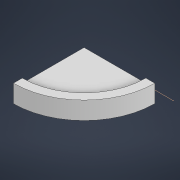
# Autodesk Inventor part: McCrea_zakruta_walle
Saved by Autodesk Inventor 2022 (Build 260153000, 153)
## iProperties
Created: 2022-02-12
Part Number: McCrea_zakruta_walle
Material: Generic
Document SubType Name: Modeling
Designer: MatusBarany
Density: 1 g/cm^3
Appearance: Default
Author: MatusBarany
Autodesk Inventor part; units mm, degrees
ref_plane "YZ Plane" through (0, 0, 0) normal (1, 0, 0) x (0, 1, 0)
ref_plane "XZ Plane" through (0, 0, 0) normal (0, 1, 0) x (-1, 0, 0)
ref_plane "XY Plane" through (0, 0, 0) normal (0, 0, 1) x (1, 0, 0)
sketch "Sketch1" plane through (0, 0, 0) normal (0, 1, 0) x (-1, 0, 0)
  arc A0 (740.7704, 834.1348) -> (40.7704, 134.1348) centre (740.7704, 134.1348) ccw
  line L0 (740.7704, 134.1348) -> (40.7704, 134.1348)
  line L1 (740.7704, 134.1348) -> (740.7704, 834.1348)
  line L2 (909.7653, 0) -> (-273.1993, 0) projected
  dimension "d2" = 1400
  constraints: 4 end point, 2 point on circle, 1 centre point, 1 parallel, 1 perpendicular
  measures "d2" diameter of A0
extrude "Extrusion1" add sketch "Sketch1" along normal blind 150
sketch "Sketch2" plane through (0, 0, 0) normal (0, -1, 0) x (1, 0, 0)
  arc A0 (-40.7704, 134.1348) -> (-740.7704, 834.1348) centre (-740.7704, 134.1348) ccw projected
  line L0 (-740.7704, 134.1348) -> (-740.7704, 834.1348) projected
  line L1 (-40.7704, 134.1348) -> (-740.7704, 134.1348) projected
  arc A1 (59.2296, 134.1348) -> (-740.7704, 934.1348) centre (-740.7704, 134.1348) ccw
  arc A2 (-40.7704, 134.1348) -> (-740.7704, 834.1348) centre (-740.7704, 134.1348) ccw projected
  line L2 (-40.7704, 134.1348) -> (59.2296, 134.1348)
  line L3 (-740.7704, 834.1348) -> (-740.7704, 934.1348)
  point P0 (0, 0)
  dimension "d5" = 100
  constraints: 4 end point, 2 point on circle, 1 centre point, 1 horizontal, 1 vertical
  measures "d5" radial gap between concentric circles of A1 A0
extrude "Extrusion2" add sketch "Sketch2" against normal blind 200 contours A0 L3 A1 L2
body "Solid1"
